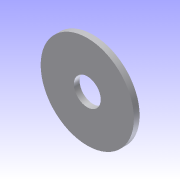
# Autodesk Inventor part: HW-00021
Saved by Autodesk Inventor 2012 (Build 160160000, 160)
## iProperties
Created: 2008-10-27
Part Number: HW-00021
Document SubType Name: Modeling
Designer: dfoster
Density: 1 g/cm^3
Description: Washer, Fender 1/4" Zinc Plate
Material: Default
Title: Washer, Fender 1/4" Zinc Plate
Author: dfoster
Autodesk Inventor part; units mm, degrees
ref_plane "YZ Plane" through (0, 0, 0) normal (1, 0, 0) x (0, 1, 0)
ref_plane "XZ Plane" through (0, 0, 0) normal (0, 1, 0) x (-1, 0, 0)
ref_plane "XY Plane" through (0, 0, 0) normal (0, 0, 1) x (1, 0, 0)
sketch "Sketch1" plane through (0, 0, 0) normal (0, 0, 1) x (1, 0, 0)
  circle A0 centre (0, 0) radius 12.7635
  circle A1 centre (0, 0) radius 3.683
  dimension "d0" = 7.366
  dimension "d1" = 25.527
  constraints: 2 centre point, 1 coincident
  measures "d0" diameter of A1
  measures "d1" diameter of A0
extrude "Extrusion1" add sketch "Sketch1" along normal blind 1.5748
body "Solid1"
